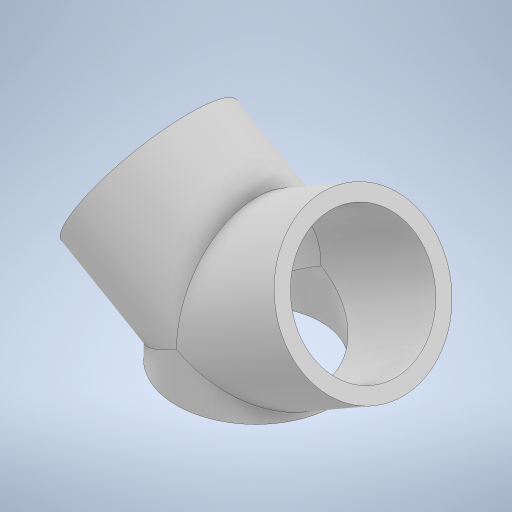
# Autodesk Inventor part: WYE-S36-SCH160-120
Saved by Autodesk Inventor 2023 (Build 270158000, 158)
## iProperties
Created: 2023-11-21
Part Number: WYE-S36-SCH160-120
Material: Generic
Document SubType Name: Modeling
Designer: Admin
Density: 1 g/cm^3
Appearance: Default
Author: Admin
Autodesk Inventor part; units mm, degrees
ref_plane "YZ Plane" through (0, 0, 0) normal (1, 0, 0) x (0, 1, 0)
sketch "Sketch1" plane through (0, 0, 0) normal (0, 0, 1) x (1, 0, 0)
  line L0 (0, 0) -> (0, 279.4)
  line L1 (0, 279.4) -> (615.9173, 635)
  line L2 (0, 279.4) -> (-615.9173, 635)
  line L3 (-615.9173, 635) -> (615.9173, 635) construction
  dimension "A_dimension" = 279.4
  dimension "angle" = 120
  dimension "B_dimension" = 711.2
  constraints: 8 end point, 1 equal length, 1 horizontal, 1 vertical
  measures "A_dimension" distance of L0.start L0.end
  measures "angle" angle of L1 L2
  measures "B_dimension" distance of L0.end L2.end
sketch "Sketch2" plane through (0, 0, 0) normal (0, 1, 0) x (-1, 0, 0)
  circle A0 centre (0, 0) radius 457.2
  circle A1 centre (0, 0) radius 373.9896
  dimension "outerDiameter" = 914.4
  dimension "wallThickness" = 83.2104
  constraints: 2 centre point, 2 coincident
  measures "outerDiameter" diameter of A0
  measures "wallThickness" radial gap between concentric circles of A0 A1
ref_plane "Work Plane1" through (615.9173, 635, 0) normal (0.8660254, 0.5, 0) x (-0.5, 0.8660254, 0)
sketch "Sketch3" plane through (615.9173, 635, 0) normal (0.8660254, 0.5, 0) x (-0.5, 0.8660254, 0)
  circle A0 centre (0, 0) radius 457.2
  circle A1 centre (0, 0) radius 373.9896
  point P0 (-241.9675, 0)
  point P1 (0, 0)
  dimension "d7" = 914.4
  dimension "d8" = 83.2104
  constraints: 2 centre point, 2 coincident
  measures "d7" diameter of A0
  measures "d8" radial gap between concentric circles of A0 A1
ref_plane "Work Plane2" through (-615.9173, 635, 0) normal (-0.8660254, 0.5, 0) x (-0.5, -0.8660254, 0)
sketch "Sketch4" plane through (-615.9173, 635, 0) normal (-0.8660254, 0.5, 0) x (-0.5, -0.8660254, 0)
  circle A0 centre (0, 0) radius 457.2
  circle A1 centre (0, 0) radius 373.9896
  point P0 (241.9675, 0)
  point P1 (0, 0)
  dimension "d9" = 914.4
  dimension "d11" = 83.2104
  constraints: 2 centre point, 2 coincident
  measures "d9" diameter of A0
  measures "d11" radial gap between concentric circles of A0 A1
extrude "Extrusion1" add sketch "Sketch2" along normal up to surface (279.4 mm away)
extrude "Extrusion2" add sketch "Sketch4" against normal up to surface (711.2 mm away)
extrude "Extrusion3" add sketch "Sketch3" against normal up to surface (711.2 mm away)
extrude "Extrusion4" cut sketch "Sketch2" along normal up to surface (279.4 mm away) contours A1
extrude "Extrusion5" cut sketch "Sketch3" against normal up to surface (711.2 mm away) contours A1
extrude "Extrusion6" cut sketch "Sketch4" against normal up to surface (711.2 mm away) contours A1
extrude "Extrusion7" cut sketch "Sketch4" along normal through all contours A0 | A1
extrude "Extrusion8" cut sketch "Sketch3" along normal through all contours A0 | A1
extrude "Extrusion9" cut sketch "Sketch2" against normal through all contours A0 | A1
equation "\"d7\" = outerDiameter"
equation "\"d8\" = wallThickness"
equation "\"d9\" = outerDiameter"
equation "\"d11\" = wallThickness"
equation "\"nominalSize\" = 914.4"
body "Solid2"
body "Solid3"
